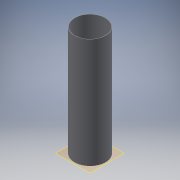
# Autodesk Inventor part: chuteback
Saved by Autodesk Inventor 2018 (Build 220112000, 112)
## iProperties
Created: 2018-02-05
Part Number: chuteback
Material: Generic
Document SubType Name: Modeling
Designer: Benedikt
Density: 1 g/cm^3
Appearance: Default
Author: Benedikt
Autodesk Inventor part; units mm, degrees
ref_plane "YZ Plane" through (0, 0, 0) normal (1, 0, 0) x (0, 1, 0)
ref_plane "XZ Plane" through (0, 0, 0) normal (0, 1, 0) x (-1, 0, 0)
ref_plane "XY Plane" through (0, 0, 0) normal (0, 0, 1) x (1, 0, 0)
ref_plane "Work Plane1" through (0, 0, 0) normal (0, 0, 1) x (1, 0, 0)
sketch "Sketch1" plane through (0, 0, 0) normal (0, 0, 1) x (1, 0, 0)
  spline S0 degree 3 poles (35.0051, -17.1191) (32.8906, -18.118) (30.893, -19.3477) (27.2046, -22.2238) (25.525, -23.8614) (21.4194, -28.8606) (19.4465, -32.534) (17.0199, -40.4304) (16.5894, -44.5779) (17.3423, -52.8043) (18.5186, -56.8047) (22.3383, -64.1294) (24.9452, -67.3836) (31.2598, -72.7098) (34.907, -74.7307) (42.7709, -77.2607) (46.9123, -77.7457) (55.1479, -77.1007) (59.1634, -75.9771) (66.5376, -72.2538) (69.8258, -69.6898) (75.2343, -63.4457) (77.3029, -59.8252) (79.9359, -51.9953) (80.4752, -47.8606) (79.9384, -39.6172) (78.8675, -35.5873) (75.2413, -28.1649) (72.7207, -24.8433) (66.5481, -19.3533) (62.9551, -17.2374) (55.1604, -14.5019) (51.0331, -13.9084) (42.7834, -14.337) (38.7398, -15.3549) (35.0051, -17.1191) knots -19.990033 -19.990033 -19.990033 -19.990033 -19.288451 -19.288451 -18.586869 -18.586869 -17.347745 -17.347745 -16.10862 -16.10862 -14.869495 -14.869495 -13.630371 -13.630371 -12.391246 -12.391246 -11.152122 -11.152122 -9.912997 -9.912997 -8.673872 -8.673872 -7.434748 -7.434748 -6.195623 -6.195623 -4.956498 -4.956498 -3.717374 -3.717374 -2.478249 -2.478249 -1.239125 -1.239125 0 0 0 0 projected
  spline S1 degree 3 poles (34.6432, -16.3055) (36.8178, -15.2799) (39.0991, -14.498) (43.7919, -13.4498) (46.1891, -13.1868) (52.8397, -13.1949) (57.0444, -14.0294) (64.8974, -17.2632) (68.4705, -19.6315) (74.5077, -25.6046) (76.9142, -29.1521) (80.2318, -36.97) (81.1112, -41.1656) (81.2123, -49.6576) (80.4331, -53.873) (77.3026, -61.7676) (74.9814, -65.3715) (69.0881, -71.4867) (65.5724, -73.9394) (57.7987, -77.3593) (53.6151, -78.2938) (45.1251, -78.5063) (40.8999, -77.7825) (32.9648, -74.7559) (29.3308, -72.4821) (23.1388, -66.6696) (20.6401, -63.1864) (17.1185, -55.4583) (16.1293, -51.2872) (15.8053, -42.8007) (16.4737, -38.5664) (19.3959, -30.5923) (21.6217, -26.9288) (27.3525, -20.6611) (30.8026, -18.1169) (34.6432, -16.3055) knots -20.551076 -20.551076 -20.551076 -20.551076 -19.829804 -19.829804 -19.108531 -19.108531 -17.834629 -17.834629 -16.560727 -16.560727 -15.286825 -15.286825 -14.012923 -14.012923 -12.739021 -12.739021 -11.465119 -11.465119 -10.191217 -10.191217 -8.917314 -8.917314 -7.643412 -7.643412 -6.36951 -6.36951 -5.095608 -5.095608 -3.821706 -3.821706 -2.547804 -2.547804 -1.273902 -1.273902 0 0 0 0 projected
  point P0 (0, 0)
  point P1 (35.0051, -17.1191)
  point P2 (34.6432, -16.3055)
extrude "Extrusion1" add sketch "Sketch1" along normal blind 230
body "Solid1"
